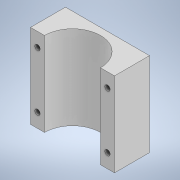
# Autodesk Inventor part: clampForMeadeTripodLeg
Saved by Autodesk Inventor 2021.2 (Build 252289000, 289)
## iProperties
Created: 2021-02-07
Part Number: clampForMeadeTripodLeg
Material: Generic
Document SubType Name: Modeling
Designer: robst
Density: 1 g/cm^3
Appearance: Default
Author: robst
Autodesk Inventor part; units mm, degrees
ref_plane "YZ Plane" through (0, 0, 0) normal (1, 0, 0) x (0, 1, 0)
ref_plane "XZ Plane" through (0, 0, 0) normal (0, 1, 0) x (-1, 0, 0)
ref_plane "XY Plane" through (0, 0, 0) normal (0, 0, 1) x (1, 0, 0)
sketch "Sketch18" plane through (0, 0, 0) normal (0, 1, 0) x (-1, 0, 0)
  arc A0 (-25.4, 0) -> (25.4, 0) centre (0, 0) ccw
  line L0 (-38.1, 0) -> (-38.1, -31.75)
  line L1 (-38.1, -31.75) -> (38.1, -31.75)
  line L2 (38.1, -31.75) -> (38.1, 0)
  line L3 (38.1, 31.75) -> (-38.1, -31.75) construction
  line L4 (-38.1, 31.75) -> (38.1, -31.75) construction
  line L5 (38.1, 0) -> (25.4, 0)
  line L6 (-25.4, 0) -> (-38.1, 0)
  dimension "d78" = 50.8
  dimension "d79" = 6.35
  dimension "d80" = 12.7
  constraints: 14 end point, 2 midpoint, 2 point on circle, 1 centre point, 1 coincident, 1 parallel
  measures "d78" diameter of A0
  measures "d79" distance edge to line of A0 L1
  measures "d80" distance edge to line of A0 L2
extrude "Extrusion9" add sketch "Sketch18" against normal blind 76.2
sketch "Sketch19" plane through (-38.1, 0, 0) normal (0, 0, 1) x (1, 0, 0)
  line L0 (0, 0) -> (0, -76.2) projected
  line L1 (12.7, 0) -> (12.7, -76.2) projected
  line L2 (63.5, 0) -> (63.5, -76.2) projected
  line L3 (76.2, 0) -> (76.2, -76.2) projected
  line L4 (76.2, -76.2) -> (63.5, -76.2) projected
  line L5 (12.7, -76.2) -> (0, -76.2) projected
  line L6 (0, 0) -> (12.7, 0) projected
  line L7 (63.5, 0) -> (76.2, 0) projected
  line L8 (6.35, -63.5) -> (69.85, -63.5) construction
  line L9 (69.85, -63.5) -> (69.85, -12.7) construction
  line L10 (69.85, -12.7) -> (6.35, -12.7) construction
  line L11 (6.35, -12.7) -> (6.35, -63.5) construction
  line L12 (63.5, -76.2) -> (12.7, -76.2) construction
  line L13 (12.7, 0) -> (63.5, 0) construction
  point P0 (38.1, 0)
  dimension "d83" = 6.35
  dimension "d84" = 6.35
  dimension "d85" = 12.7
  dimension "d86" = 12.7
  constraints: 8 end point, 4 coincident, 2 parallel, 1 horizontal, 1 perpendicular
  measures "d83" distance between parallel lines of L11 L0
  measures "d84" distance between parallel lines of L9 L3
  measures "d85" distance between parallel lines of L12 L8
  measures "d86" distance between parallel lines of L10 L13
hole "Hole3" at (-31.75, -12.7, 0) at (31.75, -12.7, 0) at (31.75, -63.5, 0) at (-31.75, -63.5, 0) direction (0, 0, -1) diameter 4.699 depth 7.1501 counterbore diameter 4.8514 counterbore depth 5.5626
sketch "Sketch20" plane through (38.1, 0, -31.75) normal (0, 0, -1) x (-1, 0, 0)
  line L0 (76.2, 0) -> (76.2, -76.2) projected
  line L1 (0, 0) -> (76.2, 0) projected
  line L2 (0, 0) -> (0, -76.2) projected
  line L3 (76.2, -76.2) -> (0, -76.2) projected
  line L4 (12.7, -63.5) -> (63.5, -63.5) construction
  line L5 (63.5, -63.5) -> (63.5, -12.7) construction
  line L6 (63.5, -12.7) -> (12.7, -12.7) construction
  line L7 (12.7, -12.7) -> (12.7, -63.5) construction
  line L8 (12.7, -63.5) -> (63.5, -12.7) construction
  line L9 (63.5, -63.5) -> (12.7, -12.7) construction
  line L10 (0, 0) -> (0, -76.2) construction
  point P0 (38.1, 0)
  point P1 (38.1, -38.1)
  dimension "d94" = 12.7
  dimension "d95" = 12.7
  dimension "d96" = 12.7
  dimension "d97" = 12.7
  constraints: 12 end point, 4 coincident, 2 midpoint, 2 parallel, 2 perpendicular
  measures "d94" distance between parallel lines of L6 L1
  measures "d95" distance between parallel lines of L4 L3
  measures "d96" distance between parallel lines of L2 L7
  measures "d97" distance between parallel lines of L0 L5
hole "Hole4" at (25.4, -12.7, -31.75) at (-25.4, -12.7, -31.75) at (-25.4, -63.5, -31.75) at (25.4, -63.5, -31.75) direction (0, 0, 1) diameter 4.7244 depth 7.1501 counterbore diameter 5.1816 counterbore depth 5.5626
sketch "Sketch21" plane through (38.1, 0, -31.75) normal (0, 0, -1) x (-1, 0, 0)
  line L0 (0, 0) -> (0, -76.2) construction
  line L1 (0, -38.1) -> (76.2, -38.1) construction
  line L2 (76.2, 0) -> (76.2, -76.2) construction
  line L3 (8.5191, -41.148) -> (4.7597, -41.148)
  line L4 (4.7597, -41.148) -> (4.7597, -40.2835)
  spline S0 degree 2 poles (4.7597, -40.2835) (5.1648, -39.9031) (5.886, -39.1967) (6.2319, -38.8163) knots 0 0 0 1 2 2 2
  spline S1 degree 2 poles (6.2319, -38.8163) (6.9284, -38.0506) (7.4372, -37.1318) (7.4372, -36.6427) knots 0 0 0 1 2 2 2
  spline S2 degree 2 poles (7.4372, -36.6427) (7.4372, -36.3858) (7.2791, -36.0005) (7.1359, -35.877) knots 0 0 0 1 2 2 2
  spline S3 degree 2 poles (7.1359, -35.877) (6.9926, -35.7535) (6.6172, -35.63) (6.3899, -35.63) knots 0 0 0 1 2 2 2
  spline S4 degree 2 poles (6.3899, -35.63) (6.1726, -35.63) (5.728, -35.7387) (5.5254, -35.8226) knots 0 0 0 1 2 2 2
  spline S5 degree 2 poles (5.5254, -35.8226) (5.3525, -35.8918) (5.0314, -36.0894) (4.9326, -36.1586) knots 0 0 0 1 2 2 2
  line L5 (4.9326, -36.1586) -> (4.8882, -36.1586)
  line L6 (4.8882, -36.1586) -> (4.8882, -35.2891)
  spline S6 degree 2 poles (4.8882, -35.2891) (5.1401, -35.1656) (6.0441, -34.9236) (6.4492, -34.9236) knots 0 0 0 1 2 2 2
  spline S7 degree 2 poles (6.4492, -34.9236) (7.3038, -34.9236) (8.2671, -35.8276) (8.2671, -36.5982) knots 0 0 0 1 2 2 2
  spline S8 degree 2 poles (8.2671, -36.5982) (8.2671, -36.9589) (8.0992, -37.5615) (7.951, -37.8184) knots 0 0 0 1 2 2 2
  spline S9 degree 2 poles (7.951, -37.8184) (7.8028, -38.0852) (7.373, -38.6088) (7.1359, -38.8608) knots 0 0 0 1 2 2 2
  spline S10 degree 2 poles (7.1359, -38.8608) (6.7506, -39.2807) (5.807, -40.1798) (5.5254, -40.4416) knots 0 0 0 1 2 2 2
  line L7 (5.5254, -40.4416) -> (8.5191, -40.4416)
  line L8 (8.5191, -40.4416) -> (8.5191, -41.148)
  line L9 (11.7894, -34.7803) -> (11.6115, -37.1515)
  line L10 (11.6115, -37.1515) -> (11.0731, -37.1515)
  line L11 (11.0731, -37.1515) -> (10.8952, -34.7803)
  line L12 (10.8952, -34.7803) -> (11.7894, -34.7803)
  line L13 (10.2481, -34.7803) -> (10.0703, -37.1515)
  line L14 (10.0703, -37.1515) -> (9.5318, -37.1515)
  line L15 (9.5318, -37.1515) -> (9.354, -34.7803)
  line L16 (9.354, -34.7803) -> (10.2481, -34.7803)
  line L17 (16.3639, -41.148) -> (15.4203, -41.148)
  line L18 (15.4203, -41.148) -> (14.3088, -39.4289)
  line L19 (14.3088, -39.4289) -> (13.1677, -41.148)
  line L20 (13.1677, -41.148) -> (12.2933, -41.148)
  line L21 (12.2933, -41.148) -> (13.879, -38.8805)
  line L22 (13.879, -38.8805) -> (12.3081, -36.5735)
  line L23 (12.3081, -36.5735) -> (13.2516, -36.5735)
  line L24 (13.2516, -36.5735) -> (14.3582, -38.2778)
  line L25 (14.3582, -38.2778) -> (15.4895, -36.5735)
  line L26 (15.4895, -36.5735) -> (16.3639, -36.5735)
  line L27 (16.3639, -36.5735) -> (14.788, -38.8311)
  line L28 (14.788, -38.8311) -> (16.3639, -41.148)
  line L29 (20.6073, -41.148) -> (16.848, -41.148)
  line L30 (16.848, -41.148) -> (16.848, -40.2835)
  spline S11 degree 2 poles (16.848, -40.2835) (17.2531, -39.9031) (17.9743, -39.1967) (18.3201, -38.8163) knots 0 0 0 1 2 2 2
  spline S12 degree 2 poles (18.3201, -38.8163) (19.0167, -38.0506) (19.5255, -37.1318) (19.5255, -36.6427) knots 0 0 0 1 2 2 2
  spline S13 degree 2 poles (19.5255, -36.6427) (19.5255, -36.3858) (19.3674, -36.0005) (19.2241, -35.877) knots 0 0 0 1 2 2 2
  spline S14 degree 2 poles (19.2241, -35.877) (19.0809, -35.7535) (18.7054, -35.63) (18.4782, -35.63) knots 0 0 0 1 2 2 2
  spline S15 degree 2 poles (18.4782, -35.63) (18.2608, -35.63) (17.8162, -35.7387) (17.6137, -35.8226) knots 0 0 0 1 2 2 2
  spline S16 degree 2 poles (17.6137, -35.8226) (17.4408, -35.8918) (17.1197, -36.0894) (17.0209, -36.1586) knots 0 0 0 1 2 2 2
  line L31 (17.0209, -36.1586) -> (16.9764, -36.1586)
  line L32 (16.9764, -36.1586) -> (16.9764, -35.2891)
  spline S17 degree 2 poles (16.9764, -35.2891) (17.2284, -35.1656) (18.1324, -34.9236) (18.5375, -34.9236) knots 0 0 0 1 2 2 2
  spline S18 degree 2 poles (18.5375, -34.9236) (19.3921, -34.9236) (20.3554, -35.8276) (20.3554, -36.5982) knots 0 0 0 1 2 2 2
  spline S19 degree 2 poles (20.3554, -36.5982) (20.3554, -36.9589) (20.1874, -37.5615) (20.0392, -37.8184) knots 0 0 0 1 2 2 2
  spline S20 degree 2 poles (20.0392, -37.8184) (19.891, -38.0852) (19.4613, -38.6088) (19.2241, -38.8608) knots 0 0 0 1 2 2 2
  spline S21 degree 2 poles (19.2241, -38.8608) (18.8388, -39.2807) (17.8953, -40.1798) (17.6137, -40.4416) knots 0 0 0 1 2 2 2
  line L33 (17.6137, -40.4416) -> (20.6073, -40.4416)
  line L34 (20.6073, -40.4416) -> (20.6073, -41.148)
  line L35 (22.3364, -34.7803) -> (22.1585, -37.1515)
  line L36 (22.1585, -37.1515) -> (21.6201, -37.1515)
  line L37 (21.6201, -37.1515) -> (21.4422, -34.7803)
  line L38 (21.4422, -34.7803) -> (22.3364, -34.7803)
  line L39 (23.8776, -34.7803) -> (23.6998, -37.1515)
  line L40 (23.6998, -37.1515) -> (23.1613, -37.1515)
  line L41 (23.1613, -37.1515) -> (22.9835, -34.7803)
  line L42 (22.9835, -34.7803) -> (23.8776, -34.7803)
  line L43 (31.1099, -41.148) -> (30.3392, -41.148)
  line L44 (30.3392, -41.148) -> (30.3392, -38.5397)
  spline S22 degree 2 poles (30.3392, -38.5397) (30.3392, -38.2235) (30.2799, -37.6801) (30.191, -37.5171) knots 0 0 0 1 2 2 2
  spline S23 degree 2 poles (30.191, -37.5171) (30.0971, -37.3442) (29.7612, -37.1762) (29.4747, -37.1762) knots 0 0 0 1 2 2 2
  spline S24 degree 2 poles (29.4747, -37.1762) (29.1882, -37.1762) (28.5806, -37.4825) (28.2891, -37.7295) knots 0 0 0 1 2 2 2
  line L45 (28.2891, -37.7295) -> (28.2891, -41.148)
  line L46 (28.2891, -41.148) -> (27.5185, -41.148)
  line L47 (27.5185, -41.148) -> (27.5185, -34.7803)
  line L48 (27.5185, -34.7803) -> (28.2891, -34.7803)
  line L49 (28.2891, -34.7803) -> (28.2891, -37.0824)
  spline S25 degree 2 poles (28.2891, -37.0824) (28.6349, -36.7711) (29.3018, -36.4451) (29.6772, -36.4451) knots 0 0 0 1 2 2 2
  spline S26 degree 2 poles (29.6772, -36.4451) (30.3491, -36.4451) (31.1099, -37.3343) (31.1099, -38.179) knots 0 0 0 1 2 2 2
  line L50 (31.1099, -38.179) -> (31.1099, -41.148)
  spline S27 degree 2 poles (35.9511, -38.8608) (35.9511, -40.0167) (34.8396, -41.2764) (33.9109, -41.2764) knots 0 0 0 1 2 2 2
  spline S28 degree 2 poles (33.9109, -41.2764) (32.9574, -41.2764) (31.8657, -39.9772) (31.8657, -38.8608) knots 0 0 0 1 2 2 2
  spline S29 degree 2 poles (31.8657, -38.8608) (31.8657, -37.7147) (32.992, -36.4451) (33.9109, -36.4451) knots 0 0 0 1 2 2 2
  spline S30 degree 2 poles (33.9109, -36.4451) (34.8396, -36.4451) (35.9511, -37.7097) (35.9511, -38.8608) knots 0 0 0 1 2 2 2
  spline S31 degree 2 poles (35.1557, -38.8608) (35.1557, -37.9716) (34.5086, -37.1071) (33.9109, -37.1071) knots 0 0 0 1 2 2 2
  spline S32 degree 2 poles (33.9109, -37.1071) (33.3131, -37.1071) (32.661, -37.9716) (32.661, -38.8608) knots 0 0 0 1 2 2 2
  spline S33 degree 2 poles (32.661, -38.8608) (32.661, -39.7253) (33.3131, -40.6145) (33.9109, -40.6145) knots 0 0 0 1 2 2 2
  spline S34 degree 2 poles (33.9109, -40.6145) (34.5037, -40.6145) (35.1557, -39.7401) (35.1557, -38.8608) knots 0 0 0 1 2 2 2
  line L51 (37.527, -41.148) -> (36.7563, -41.148)
  line L52 (36.7563, -41.148) -> (36.7563, -34.7803)
  line L53 (36.7563, -34.7803) -> (37.527, -34.7803)
  line L54 (37.527, -34.7803) -> (37.527, -41.148)
  spline S35 degree 2 poles (40.6441, -41.2517) (39.5474, -41.2517) (38.3421, -40.0217) (38.3421, -38.8855) knots 0 0 0 1 2 2 2
  spline S36 degree 2 poles (38.3421, -38.8855) (38.3421, -37.769) (39.5128, -36.4451) (40.4564, -36.4451) knots 0 0 0 1 2 2 2
  spline S37 degree 2 poles (40.4564, -36.4451) (40.8812, -36.4451) (41.5383, -36.6921) (41.7803, -36.9539) knots 0 0 0 1 2 2 2
  spline S38 degree 2 poles (41.7803, -36.9539) (42.0273, -37.2157) (42.2891, -37.9716) (42.2891, -38.5199) knots 0 0 0 1 2 2 2
  line L55 (42.2891, -38.5199) -> (42.2891, -38.9398)
  line L56 (42.2891, -38.9398) -> (39.1226, -38.9398)
  spline S39 degree 2 poles (39.1226, -38.9398) (39.1226, -39.7352) (39.9229, -40.5799) (40.6342, -40.5799) knots 0 0 0 1 2 2 2
  spline S40 degree 2 poles (40.6342, -40.5799) (40.8862, -40.5799) (41.3752, -40.4663) (41.5728, -40.3774) knots 0 0 0 1 2 2 2
  spline S41 degree 2 poles (41.5728, -40.3774) (41.7803, -40.2786) (42.0668, -40.1057) (42.1607, -40.0266) knots 0 0 0 1 2 2 2
  line L57 (42.1607, -40.0266) -> (42.2052, -40.0266)
  line L58 (42.2052, -40.0266) -> (42.2052, -40.8664)
  spline S42 degree 2 poles (42.2052, -40.8664) (42.0718, -40.9208) (41.6667, -41.0788) (41.5086, -41.1233) knots 0 0 0 1 2 2 2
  spline S43 degree 2 poles (41.5086, -41.1233) (41.2863, -41.1875) (40.9208, -41.2517) (40.6441, -41.2517) knots 0 0 0 1 2 2 2
  spline S44 degree 2 poles (41.5383, -38.3519) (41.5284, -38.0407) (41.3999, -37.5862) (41.2764, -37.4331) knots 0 0 0 1 2 2 2
  spline S45 degree 2 poles (41.2764, -37.4331) (41.1431, -37.2602) (40.7232, -37.0774) (40.4119, -37.0774) knots 0 0 0 1 2 2 2
  spline S46 degree 2 poles (40.4119, -37.0774) (40.1057, -37.0774) (39.6759, -37.2602) (39.498, -37.438) knots 0 0 0 1 2 2 2
  spline S47 degree 2 poles (39.498, -37.438) (39.3251, -37.6208) (39.1473, -38.0605) (39.1226, -38.3519) knots 0 0 0 1 2 2 2
  line L59 (39.1226, -38.3519) -> (41.5383, -38.3519)
  spline S48 degree 2 poles (49.5214, -38.7373) (49.5214, -39.8834) (48.4296, -41.2369) (47.5947, -41.2369) knots 0 0 0 1 2 2 2
  spline S49 degree 2 poles (47.5947, -41.2369) (47.2539, -41.2369) (46.7302, -41.0788) (46.4585, -40.9158) knots 0 0 0 1 2 2 2
  line L60 (46.4585, -40.9158) -> (46.4585, -42.8326)
  line L61 (46.4585, -42.8326) -> (45.6879, -42.8326)
  line L62 (45.6879, -42.8326) -> (45.6879, -36.5735)
  line L63 (45.6879, -36.5735) -> (46.4585, -36.5735)
  line L64 (46.4585, -36.5735) -> (46.4585, -37.0527)
  spline S50 degree 2 poles (46.4585, -37.0527) (46.7451, -36.7909) (47.4465, -36.4451) (47.8566, -36.4451) knots 0 0 0 1 2 2 2
  spline S51 degree 2 poles (47.8566, -36.4451) (48.642, -36.4451) (49.5214, -37.69) (49.5214, -38.7373) knots 0 0 0 1 2 2 2
  spline S52 degree 2 poles (48.726, -38.8262) (48.726, -38.0407) (48.2271, -37.1762) (47.6688, -37.1762) knots 0 0 0 1 2 2 2
  spline S53 degree 2 poles (47.6688, -37.1762) (47.3428, -37.1762) (46.7302, -37.4677) (46.4585, -37.6949) knots 0 0 0 1 2 2 2
  line L65 (46.4585, -37.6949) -> (46.4585, -40.2934)
  spline S54 degree 2 poles (46.4585, -40.2934) (46.7599, -40.4366) (47.1897, -40.5453) (47.4663, -40.5453) knots 0 0 0 1 2 2 2
  spline S55 degree 2 poles (47.4663, -40.5453) (48.064, -40.5453) (48.726, -39.666) (48.726, -38.8262) knots 0 0 0 1 2 2 2
  spline S56 degree 2 poles (52.8707, -40.6639) (52.7768, -40.733) (52.4607, -40.98) (52.3125, -41.0541) knots 0 0 0 1 2 2 2
  spline S57 degree 2 poles (52.3125, -41.0541) (52.1099, -41.1628) (51.7295, -41.2764) (51.3837, -41.2764) knots 0 0 0 1 2 2 2
  spline S58 degree 2 poles (51.3837, -41.2764) (51.1022, -41.2764) (50.5933, -41.064) (50.4007, -40.8714) knots 0 0 0 1 2 2 2
  spline S59 degree 2 poles (50.4007, -40.8714) (50.2179, -40.6836) (49.9956, -40.1304) (49.9956, -39.8241) knots 0 0 0 1 2 2 2
  spline S60 degree 2 poles (49.9956, -39.8241) (49.9956, -39.3498) (50.3957, -38.678) (50.8305, -38.4853) knots 0 0 0 1 2 2 2
  spline S61 degree 2 poles (50.8305, -38.4853) (51.2158, -38.3075) (52.2631, -38.1741) (52.8707, -38.1395) knots 0 0 0 1 2 2 2
  line L66 (52.8707, -38.1395) -> (52.8707, -37.9913)
  spline S62 degree 2 poles (52.8707, -37.9913) (52.8707, -37.7246) (52.7077, -37.3936) (52.5595, -37.2997) knots 0 0 0 1 2 2 2
  spline S63 degree 2 poles (52.5595, -37.2997) (52.4113, -37.2059) (51.9864, -37.1466) (51.7592, -37.1466) knots 0 0 0 1 2 2 2
  spline S64 degree 2 poles (51.7592, -37.1466) (51.4924, -37.1466) (50.7712, -37.3047) (50.4106, -37.4578) knots 0 0 0 1 2 2 2
  line L67 (50.4106, -37.4578) -> (50.3661, -37.4578)
  line L68 (50.3661, -37.4578) -> (50.3661, -36.6723)
  spline S65 degree 2 poles (50.3661, -36.6723) (50.5785, -36.6131) (51.3739, -36.4648) (51.7641, -36.4648) knots 0 0 0 1 2 2 2
  spline S66 degree 2 poles (51.7641, -36.4648) (52.2384, -36.4648) (52.8855, -36.6131) (53.1424, -36.8057) knots 0 0 0 1 2 2 2
  spline S67 degree 2 poles (53.1424, -36.8057) (53.3943, -36.9934) (53.6413, -37.5912) (53.6413, -38.021) knots 0 0 0 1 2 2 2
  line L69 (53.6413, -38.021) -> (53.6413, -41.148)
  line L70 (53.6413, -41.148) -> (52.8707, -41.148)
  line L71 (52.8707, -41.148) -> (52.8707, -40.6639)
  line L72 (52.8707, -40.0217) -> (52.8707, -38.7521)
  spline S68 degree 2 poles (52.8707, -38.7521) (52.5941, -38.7768) (51.7592, -38.8608) (51.4974, -38.9398) knots 0 0 0 1 2 2 2
  spline S69 degree 2 poles (51.4974, -38.9398) (51.1911, -39.0337) (50.7909, -39.4239) (50.7909, -39.7697) knots 0 0 0 1 2 2 2
  spline S70 degree 2 poles (50.7909, -39.7697) (50.7909, -40.1649) (51.2355, -40.5651) (51.6604, -40.5651) knots 0 0 0 1 2 2 2
  spline S71 degree 2 poles (51.6604, -40.5651) (52.021, -40.5651) (52.6138, -40.2539) (52.8707, -40.0217) knots 0 0 0 1 2 2 2
  spline S72 degree 2 poles (56.1064, -41.2369) (55.479, -41.2369) (54.7726, -40.5206) (54.7726, -39.745) knots 0 0 0 1 2 2 2
  line L73 (54.7726, -39.745) -> (54.7726, -37.2108)
  line L74 (54.7726, -37.2108) -> (54.2539, -37.2108)
  line L75 (54.2539, -37.2108) -> (54.2539, -36.5735)
  line L76 (54.2539, -36.5735) -> (54.7726, -36.5735)
  line L77 (54.7726, -36.5735) -> (54.7726, -35.2595)
  line L78 (54.7726, -35.2595) -> (55.5433, -35.2595)
  line L79 (55.5433, -35.2595) -> (55.5433, -36.5735)
  line L80 (55.5433, -36.5735) -> (56.961, -36.5735)
  line L81 (56.961, -36.5735) -> (56.961, -37.2108)
  line L82 (56.961, -37.2108) -> (55.5433, -37.2108)
  line L83 (55.5433, -37.2108) -> (55.5433, -39.3893)
  spline S73 degree 2 poles (55.5433, -39.3893) (55.5433, -39.7352) (55.568, -40.1155) (55.6519, -40.2786) knots 0 0 0 1 2 2 2
  spline S74 degree 2 poles (55.6519, -40.2786) (55.7211, -40.4218) (56.0323, -40.5651) (56.2991, -40.5651) knots 0 0 0 1 2 2 2
  spline S75 degree 2 poles (56.2991, -40.5651) (56.4868, -40.5651) (56.8375, -40.4515) (56.9166, -40.4169) knots 0 0 0 1 2 2 2
  line L84 (56.9166, -40.4169) -> (56.961, -40.4169)
  line L85 (56.961, -40.4169) -> (56.961, -41.1085)
  spline S76 degree 2 poles (56.961, -41.1085) (56.7437, -41.1678) (56.2991, -41.2369) (56.1064, -41.2369) knots 0 0 0 1 2 2 2
  spline S77 degree 2 poles (58.9124, -41.2369) (58.285, -41.2369) (57.5785, -40.5206) (57.5785, -39.745) knots 0 0 0 1 2 2 2
  line L86 (57.5785, -39.745) -> (57.5785, -37.2108)
  line L87 (57.5785, -37.2108) -> (57.0598, -37.2108)
  line L88 (57.0598, -37.2108) -> (57.0598, -36.5735)
  line L89 (57.0598, -36.5735) -> (57.5785, -36.5735)
  line L90 (57.5785, -36.5735) -> (57.5785, -35.2595)
  line L91 (57.5785, -35.2595) -> (58.3492, -35.2595)
  line L92 (58.3492, -35.2595) -> (58.3492, -36.5735)
  line L93 (58.3492, -36.5735) -> (59.767, -36.5735)
  line L94 (59.767, -36.5735) -> (59.767, -37.2108)
  line L95 (59.767, -37.2108) -> (58.3492, -37.2108)
  line L96 (58.3492, -37.2108) -> (58.3492, -39.3893)
  spline S78 degree 2 poles (58.3492, -39.3893) (58.3492, -39.7352) (58.3739, -40.1155) (58.4579, -40.2786) knots 0 0 0 1 2 2 2
  spline S79 degree 2 poles (58.4579, -40.2786) (58.527, -40.4218) (58.8383, -40.5651) (59.105, -40.5651) knots 0 0 0 1 2 2 2
  spline S80 degree 2 poles (59.105, -40.5651) (59.2927, -40.5651) (59.6435, -40.4515) (59.7225, -40.4169) knots 0 0 0 1 2 2 2
  line L97 (59.7225, -40.4169) -> (59.767, -40.4169)
  line L98 (59.767, -40.4169) -> (59.767, -41.1085)
  spline S81 degree 2 poles (59.767, -41.1085) (59.5496, -41.1678) (59.105, -41.2369) (58.9124, -41.2369) knots 0 0 0 1 2 2 2
  spline S82 degree 2 poles (62.321, -41.2517) (61.2243, -41.2517) (60.0189, -40.0217) (60.0189, -38.8855) knots 0 0 0 1 2 2 2
  spline S83 degree 2 poles (60.0189, -38.8855) (60.0189, -37.769) (61.1897, -36.4451) (62.1333, -36.4451) knots 0 0 0 1 2 2 2
  spline S84 degree 2 poles (62.1333, -36.4451) (62.5581, -36.4451) (63.2151, -36.6921) (63.4572, -36.9539) knots 0 0 0 1 2 2 2
  spline S85 degree 2 poles (63.4572, -36.9539) (63.7042, -37.2157) (63.966, -37.9716) (63.966, -38.5199) knots 0 0 0 1 2 2 2
  line L99 (63.966, -38.5199) -> (63.966, -38.9398)
  line L100 (63.966, -38.9398) -> (60.7994, -38.9398)
  spline S86 degree 2 poles (60.7994, -38.9398) (60.7994, -39.7352) (61.5997, -40.5799) (62.3111, -40.5799) knots 0 0 0 1 2 2 2
  spline S87 degree 2 poles (62.3111, -40.5799) (62.563, -40.5799) (63.0521, -40.4663) (63.2497, -40.3774) knots 0 0 0 1 2 2 2
  spline S88 degree 2 poles (63.2497, -40.3774) (63.4572, -40.2786) (63.7437, -40.1057) (63.8376, -40.0266) knots 0 0 0 1 2 2 2
  line L101 (63.8376, -40.0266) -> (63.882, -40.0266)
  line L102 (63.882, -40.0266) -> (63.882, -40.8664)
  spline S89 degree 2 poles (63.882, -40.8664) (63.7486, -40.9208) (63.3436, -41.0788) (63.1855, -41.1233) knots 0 0 0 1 2 2 2
  spline S90 degree 2 poles (63.1855, -41.1233) (62.9632, -41.1875) (62.5976, -41.2517) (62.321, -41.2517) knots 0 0 0 1 2 2 2
  spline S91 degree 2 poles (63.2151, -38.3519) (63.2052, -38.0407) (63.0768, -37.5862) (62.9533, -37.4331) knots 0 0 0 1 2 2 2
  spline S92 degree 2 poles (62.9533, -37.4331) (62.8199, -37.2602) (62.4, -37.0774) (62.0888, -37.0774) knots 0 0 0 1 2 2 2
  spline S93 degree 2 poles (62.0888, -37.0774) (61.7825, -37.0774) (61.3527, -37.2602) (61.1749, -37.438) knots 0 0 0 1 2 2 2
  spline S94 degree 2 poles (61.1749, -37.438) (61.002, -37.6208) (60.8241, -38.0605) (60.7994, -38.3519) knots 0 0 0 1 2 2 2
  line L103 (60.7994, -38.3519) -> (63.2151, -38.3519)
  line L104 (67.1721, -37.3985) -> (67.1326, -37.3985)
  spline S95 degree 2 poles (67.1326, -37.3985) (67.0437, -37.3738) (66.851, -37.3639) (66.7176, -37.3639) knots 0 0 0 1 2 2 2
  spline S96 degree 2 poles (66.7176, -37.3639) (66.4064, -37.3639) (65.7938, -37.6356) (65.5172, -37.9024) knots 0 0 0 1 2 2 2
  line L105 (65.5172, -37.9024) -> (65.5172, -41.148)
  line L106 (65.5172, -41.148) -> (64.7465, -41.148)
  line L107 (64.7465, -41.148) -> (64.7465, -36.5735)
  line L108 (64.7465, -36.5735) -> (65.5172, -36.5735)
  line L109 (65.5172, -36.5735) -> (65.5172, -37.2553)
  spline S97 degree 2 poles (65.5172, -37.2553) (65.9371, -36.8798) (66.5645, -36.5735) (66.8609, -36.5735) knots 0 0 0 1 2 2 2
  spline S98 degree 2 poles (66.8609, -36.5735) (66.9794, -36.5735) (67.098, -36.5834) (67.1721, -36.5982) knots 0 0 0 1 2 2 2
  line L110 (67.1721, -36.5982) -> (67.1721, -37.3985)
  line L111 (71.3612, -41.148) -> (70.5906, -41.148)
  line L112 (70.5906, -41.148) -> (70.5906, -38.5397)
  spline S99 degree 2 poles (70.5906, -38.5397) (70.5906, -38.2235) (70.5313, -37.6801) (70.4424, -37.5171) knots 0 0 0 1 2 2 2
  spline S100 degree 2 poles (70.4424, -37.5171) (70.3485, -37.3442) (70.0126, -37.1762) (69.7261, -37.1762) knots 0 0 0 1 2 2 2
  spline S101 degree 2 poles (69.7261, -37.1762) (69.4396, -37.1762) (68.8319, -37.4825) (68.5405, -37.7295) knots 0 0 0 1 2 2 2
  line L113 (68.5405, -37.7295) -> (68.5405, -41.148)
  line L114 (68.5405, -41.148) -> (67.7698, -41.148)
  line L115 (67.7698, -41.148) -> (67.7698, -36.5735)
  line L116 (67.7698, -36.5735) -> (68.5405, -36.5735)
  line L117 (68.5405, -36.5735) -> (68.5405, -37.0824)
  spline S102 degree 2 poles (68.5405, -37.0824) (68.8863, -36.7711) (69.5532, -36.4451) (69.9286, -36.4451) knots 0 0 0 1 2 2 2
  spline S103 degree 2 poles (69.9286, -36.4451) (70.6005, -36.4451) (71.3612, -37.3343) (71.3612, -38.179) knots 0 0 0 1 2 2 2
  line L118 (71.3612, -38.179) -> (71.3612, -41.148)
  point P0 (38.1, 0)
  constraints: 2 end point, 2 midpoint, 1 horizontal
extrude "Extrusion10" cut sketch "Sketch21" against normal blind 1.27
equation "\"d78\" = legDiameter"
equation "\"d81\" = legPartHeight"
equation "\"d98\" = diameterOfBottomOfHeatInsert"
equation "\"d100\" = diameterOfTopOfHeatInsert"
equation "\"d101\" = heitghtOfTopOfHeatInsert"
equation "\"d103\" = heightOfBottomOfHeatInsert"
equation "\"legDiameter\" = 50.8"
equation "\"legWalThickness\" = 3.175"
equation "\"legPartHeight\" = 76.2"
equation "\"heightOfBottomOfHeatInsert\" = 1.5875"
equation "\"heitghtOfTopOfHeatInsert\" = 5.5626"
equation "\"diameterOfBottomOfHeatInsert\" = 4.7244"
equation "\"diameterOfTopOfHeatInsert\" = 5.1816"
equation "\"heightOfInsert\" = heightOfBottomOfHeatInsert + heitghtOfTopOfHeatInsert"
body "Solid1"
body "Solid2"
